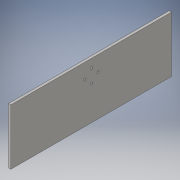
# Autodesk Inventor part: FlatPlow
Saved by Autodesk Inventor 2016 (Build 200138000, 138)
## iProperties
Created: 2016-12-19
Part Number: FlatPlow
Material: Generic
Document SubType Name: Modeling
Designer: lachesis
Density: 1 g/cm^3
Appearance: Default
Author: lachesis
Autodesk Inventor part; units mm, degrees
ref_plane "YZ Plane" through (0, 0, 0) normal (1, 0, 0) x (0, 1, 0)
ref_plane "XZ Plane" through (0, 0, 0) normal (0, 1, 0) x (-1, 0, 0)
ref_plane "XY Plane" through (0, 0, 0) normal (0, 0, 1) x (1, 0, 0)
sketch "Sketch1" plane through (0, 0, 0) normal (1, 0, 0) x (0, 1, 0)
  line L0 (35, 100.7745) -> (-35, 100.7745)
  line L1 (-35, 100.7745) -> (-35, -100.7745)
  line L2 (-35, -100.7745) -> (35, -100.7745)
  line L3 (35, -100.7745) -> (35, 100.7745)
  point P0 (0, 0)
  point P1 (0, 100.7745)
  point P2 (35, 0)
  dimension "d0" = 201.549
  dimension "d1" = 70
  constraints: 8 end point, 2 midpoint, 2 parallel, 1 horizontal, 1 horizontal alignment, 1 perpendicular, 1 vertical alignment
  measures "d0" distance of L2.end L0.start
  measures "d1" distance of L0.start L0.end
extrude "Extrusion1" add sketch "Sketch1" along normal blind 3
sketch "Sketch2" plane through (3, 0, 0) normal (1, 0, 0) x (0, 0, -1)
  circle A0 centre (0, 24.531) radius 1.345
  circle A1 centre (0, 7.869) radius 1.345
  circle A2 centre (8.331, 16.2) radius 1.345
  circle A3 centre (-8.331, 16.2) radius 1.345
  line L0 (-100.7745, 35) -> (-100.7745, -35) projected
  line L1 (-100.7745, -35) -> (100.7745, -35) projected
  line L2 (100.7745, -35) -> (100.7745, 35) projected
  line L3 (100.7745, 35) -> (-100.7745, 35) projected
  point P0 (0, 0)
  dimension "d4" = 2.69
  dimension "d10" = 10.469
  dimension "d13" = 8.331
  dimension "d14" = 8.331
  dimension "d15" = 8.331
  dimension "d16" = 8.331
  dimension "d17" = 16.662
  dimension "d18" = 16.662
  constraints: 4 centre point, 3 equal radius, 1 vertical alignment
  measures "d4" diameter of A0
  measures "d10" distance from line of A0.centre L3
  measures "d13" horizontal distance of A2.centre A0.centre
  measures "d14" horizontal distance of A1.centre A3.centre
  measures "d15" horizontal distance of A0.centre A3.centre
  measures "d16" horizontal distance of A2.centre A1.centre
  measures "d17" distance of A1.centre A0.centre
  measures "d18" distance of A2.centre A3.centre
extrude "Extrusion2" cut sketch "Sketch2" against normal through all contours A0 | A1 | A2 | A3
equation "\"d14\" = d13"
equation "\"d15\" = d13"
equation "\"d16\" = d13"
equation "\"d18\" = d17"
body "Solid1"
